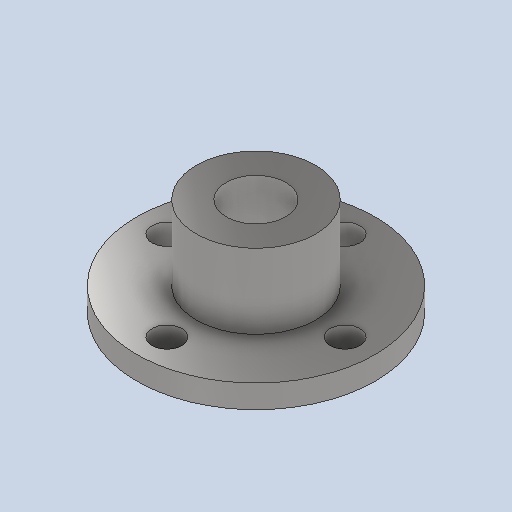
# Autodesk Inventor part: FlangeCoupling
Saved by Autodesk Inventor 2022.2 (Build 262287000, 287)
## iProperties
Created: 2022-07-30
Part Number: FlangeCoupling
Material: Steel, Mild
Document SubType Name: Modeling
Designer: ABL
Density: 7.85 g/cm^3
Appearance: Semi-Polished
Author: ABL
Autodesk Inventor part; units mm, degrees
ref_plane "YZ Plane" through (0, 0, 0) normal (1, 0, 0) x (0, 1, 0)
ref_plane "XZ Plane" through (0, 0, 0) normal (0, 1, 0) x (-1, 0, 0)
ref_plane "XY Plane" through (0, 0, 0) normal (0, 0, 1) x (1, 0, 0)
sketch "Sketch1" plane through (0, 0, 0) normal (0, 0, 1) x (1, 0, 0)
  line L0 (0, 0) -> (0, 13.1) construction
  line L1 (4, 0) -> (4, 13.1)
  line L2 (4, 13.1) -> (8, 13.1)
  line L3 (8, 13.1) -> (8, 3.1)
  line L4 (8, 3.1) -> (16, 3.1)
  line L5 (16, 3.1) -> (16, 0)
  line L6 (16, 0) -> (4, 0)
  point P0 (8, 8.1)
  point P1 (8, 8.1)
  dimension "d0" = 13.1
  dimension "d1" = 10
  dimension "d2" = 3.1
  dimension "d3" = 32
  dimension "d4" = 16
  dimension "d5" = 8
  constraints: 14 end point, 5 perpendicular, 2 vertical, 1 coincident, 1 midpoint
  measures "d0" distance of L0.start L0.end
  measures "d1" distance of L2.end L3.end
  measures "d2" distance of L4.end L5.end
  measures "d3" diameter of L5 L0
  measures "d4" diameter of L3 L0
  measures "d5" diameter of L1 L0
revolve "Revolution1" add sketch "Sketch1" angle 360 about axis through (0, 0, 0) along (0, 1, 0)
sketch "Sketch2" plane through (0, 0, 0) normal (0, -1, 0) x (1, 0, 0)
  circle A0 centre (11.95, 0) radius 2
  line L0 (13.95, 0) -> (16, 0) construction
  circle A1 centre (0, 0) radius 16 construction
  dimension "d7" = 4
  dimension "d8" = 2.05
  constraints: 2 end point, 2 horizontal alignment, 3 other
  measures "d8" distance of L0.start L0.end
extrude "MountHole" cut sketch "Sketch2" against normal through all
pattern_circular "Circular Pattern1" count 4 over 360 about axis through (0, 6.55, 0) along (0, -1, 0) of "MountHole"
equation "\"d0\" = flangeCoupling_height"
equation "\"d1\" = flangeCoupling_collarHeight"
equation "\"d2\" = flangeCoupling_flangeHeight"
equation "\"d3\" = flangeCoupling_flangeDiameter"
equation "\"d4\" = flangeCoupling_collarOuterDiameter"
equation "\"d5\" = flangeCoupling_innerDiameter"
equation "\"d7\" = flangeCoupling_mountHoleDiameter + gap"
equation "\"d8\" = flangeCoupling_mountHoleEdgeToEdge"
equation "\"gap\" = 0.1"
equation "\"airgap\" = 0.4"
equation "\"wallgap\" = 2"
equation "\"driveMagnet_height\" = 5"
equation "\"halbachMagnet_height\" = 3"
equation "\"rotorBandBolt_diameter\" = 2"
equation "\"rotorBandBolt_headDiameter\" = 3.98"
equation "\"rotorBandBolt_headHeight\" = 2"
equation "\"rotorBandHexNut_sideToSide\" = 4"
equation "\"rotorBandHexNut_height\" = 1.2"
equation "\"rotorBandSquareNut_sideLength\" = 4"
equation "\"rotorBandSquareNut_height\" = 1.2"
equation "\"sensorMagnet_diameter\" = 5"
equation "\"sensorMagnet_height\" = 2.66667"
equation "\"rotorRadius\" = 2 * gap + driveMagnet_centerSpacingRadius + driveMagnet_length + wallgap"
equation "\"rotor_mountingLipHeight\" = 0.5 * statorThickness"
equation "\"shaftDiameter\" = 8"
equation "\"flangeBearing_innerDiameter\" = shaftDiameter"
equation "\"flangeBearing_outerDiameter\" = 16"
equation "\"flangeBearing_flangeDiameter\" = 18"
equation "\"flangeBearing_height\" = 5"
equation "\"flangeBearing_flangeHeight\" = 1"
equation "\"statorThickness\" = coilThickness + 2 * wallgap"
equation "\"rotorBandThickness\" = wallgap + rotorBandBolt_headHeight + gap"
equation "\"flangeCoupling_innerDiameter\" = shaftDiameter"
equation "\"flangeCoupling_collarOuterDiameter\" = 16"
equation "\"flangeCoupling_flangeDiameter\" = 32"
equation "\"flangeCoupling_collarHeight\" = 10"
equation "\"flangeCoupling_flangeHeight\" = 3.1"
equation "\"flangeCoupling_flangeHoleDiameter\" = 3.9"
equation "\"flangeCoupling_flangeHoleEdgeToEdge\" = 2.05"
equation "\"flangeCoupling_height\" = flangeCoupling_collarHeight + flangeCoupling_flangeHeight"
equation "\"flangeCoupling_mountHoleDiameter\" = 3.9"
equation "\"flangeCoupling_mountHoleEdgeToEdge\" = 2.05"
equation "\"statorRadius\" = driveMagnet_length + driveMagnet_centerSpacingRadius + 2 * gap"
equation "\"coilThickness\" = 12"
equation "\"statorMountBolt_diameter\" = 4"
equation "\"statorMountBolt_headDiameter\" = 7"
equation "\"statorMountBolt_headHeight\" = 4"
equation "\"statorMountBolt_shaftLength\" = coilThickness + flangeCoupling_flangeHeight + wallgap"
equation "\"statorMountHexNut_height\" = 4"
equation "\"statorMountHexNut_sideToSide\" = 8"
equation "\"sensorMagnet_ringRadius\" = 0.5 * driveMagnet_centerSpacingRadius + 2 * wallgap"
equation "\"coil_percentCoverage\" = 0.6"
equation "\"statorSpokeDegrees\" = 4deg"
equation "\"coil_bulge\" = 3"
equation "\"statorCoilBolt_shaftLength\" = coilThickness"
equation "\"statorCoilHexNut_height\" = 1.2"
equation "\"statorCoilBolt_headHeight\" = 2"
equation "\"statorCoilBolt_diameter\" = 2"
equation "\"statorCoilBolt_headDiameter\" = 3.98"
equation "\"statorCoilHexNut_sideToSide\" = 4"
equation "\"magnetWire_outerDiameter\" = 0.8128"
equation "\"printingLayerHeight\" = 0.2"
equation "\"circuitBoard_height\" = 1.6"
equation "\"hallEffectSensor_width\" = 1.6"
equation "\"hallEffectSensor_length\" = 3"
equation "\"hallEffectSensor_height\" = 1.1"
equation "\"hallEffectSensor_pinLength\" = 0.6"
equation "\"circuitboardMountHexNut_height\" = 1.2"
equation "\"circuitboardMountHexNut_sideToSide\" = 4"
equation "\"circuitboardMountBolt_headHeight\" = 2"
equation "\"circuitboardMountBolt_shaftLength\" = coilThickness"
equation "\"circuitboardMountBolt_diameter\" = 2"
equation "\"circuitboardMountBolt_headDiameter\" = 3.98"
equation "\"statorShellBolt_headDiameter\" = 5.68"
equation "\"statorShellHexNut_height\" = 2.3"
equation "\"statorShellBolt_shaftLength\" = statorThickness - statorShellBolt_countersinkDepth"
equation "\"statorShellBolt_headHeight\" = 3"
equation "\"statorShellHexNut_sideToSide\" = 5.3"
equation "\"statorShellBolt_diameter\" = 3"
equation "\"driveMagnet_centerSpacingRadius\" = 38.96113"
equation "\"driveMagnet_length\" = 60"
equation "\"statorShellBolt_countersinkDepth\" = 3.4"
